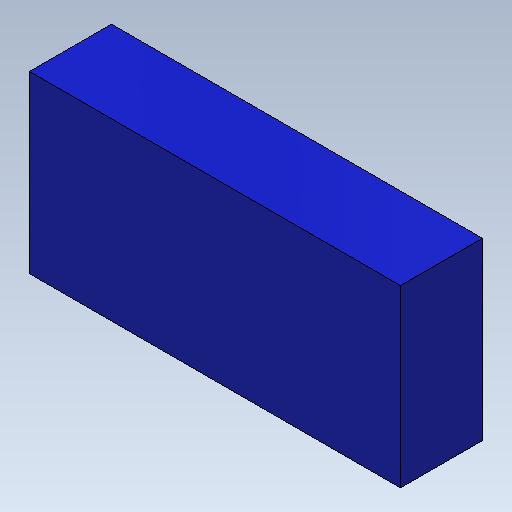
# Autodesk Inventor part: LTP
Saved by Autodesk Inventor 2020.1 (Build 241239000, 239)
## iProperties
Part Number: LTP
Document SubType Name: Modeling
Created: 2003-10-21
Designer: brondec
Manufacturer: Standard
Standards Organization: Custom
Density: 1 g/cm^3
Mass: 1.13797 g
Surface Area: 7.79089 cm^2
Volume: 1.13797 cm^3
Material: Generic
Appearance: Blue - Wall Paint - Glossy
Control State: 0
Master: False
Checked Out: False
Shininess: 64.0
Length Units: 11272
Angle Units: 11279
Time Units: 11290
Mass Units: 11286
Length Display Precision: 3
Angle Display Precision: 2
Compacted: True
Density: 0.0
Volumn: 0.0
Area: 0.0
PropertySet Name: Model Information
Author: brondec
Autodesk Inventor part; units mm, degrees
ref_plane "YZ Plane" through (0, 0, 0) normal (1, 0, 0) x (0, 1, 0)
ref_plane "XZ Plane" through (0, 0, 0) normal (0, 1, 0) x (-1, 0, 0)
ref_plane "XY Plane" through (0, 0, 0) normal (0, 0, 1) x (1, 0, 0)
sketch "Sketch3" plane through (0, 0, 0) normal (0, 0, 1) x (1, 0, 0)
  line L0 (0.9525, -1.651) -> (13.6525, -1.651)
  line L1 (13.6525, -1.651) -> (13.6525, 4.3434)
  line L2 (13.6525, 4.3434) -> (0.9525, 4.3434)
  line L3 (0.9525, 4.3434) -> (0.9525, -1.651)
  point P0 (0, 0)
  dimension "d17" = 5.9944
  dimension "d18" = 12.7
  dimension "d19" = 0.9525
  dimension "d20" = 1.651
  constraints: 8 end point, 2 parallel, 1 horizontal, 1 perpendicular
  measures "d17" distance of L2.end L0.start
  measures "d18" distance of L1.end L2.end
  measures "d19" distance from line of L3 point (0, 0)
  measures "d20" distance from line of point (0, 0) L0
extrude "Extrusion1" add sketch "Sketch3" along normal blind 2.8067
body "Solid1"
